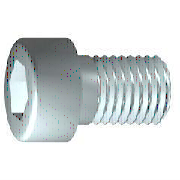
# Autodesk Inventor part: 100021
Saved by Autodesk Inventor 2020.1 (Build 241239000, 239)
## iProperties
Created: 2006-01-26
Part Number: 100021
Material: Steel, Mild
Description: Hexagon Socket Head Cap Screw
Vendor: Autodesk Inc.
Document SubType Name: Modeling
Standard: ISO 4762
Designer: Kevin
Standard Revision: Fourth edition 2004-03-01
Standards Organization: ISO
Language: en-US
Size Designation: M8 x 65
Categories: <MemberInstance><Categories><Category DisplayName="Fasteners" InternalName="e4da775c-781d-43d5-af7c-5136215cf5a6" Mnemonic="FSTN"><Category DisplayName="Bolts" InternalName="536e6df0-f778-49ac-b2f2-25c71d2aa0b2" Mnemonic="SCRW"><CategoryParameter DisplayName="Nominal Diameter" InternalName="8bbe3f8e-44cf-40a9-a251-3a6edc8168d6" Mnemonic="nomdia"/><CategoryParameter DisplayName="Nominal Length" InternalName="238ecbaf-3e6c-45dd-aa95-4068c8e0fd02" Mnemonic="nomlen"/><CategoryParameter DisplayName="Thread Series Designation" InternalName="87c5849c-b3a5-4c3e-9c9b-2feecef9be86" Mnemonic="thrserdsgn"/><CategoryParameter DisplayName="Thread Class" InternalName="ebc0d23b-2cc6-4d2a-b376-d52aae53bab6" Mnemonic="thrclss"/><CategoryParameter DisplayName="Thread Designation" InternalName="586d5e89-370a-4089-914f-0110033585c7" Mnemonic="thrdesign"/><CategoryParameter DisplayName="Thread Type" InternalName="b4bbb7bc-d6aa-4c9f-a9a9-4152b9f6fe49" Mnemonic="thrtype"/><CategoryParameter DisplayName="Threads per Unit" InternalName="bdc6e7d2-ffd0-4d9c-a173-16b95ebb912d" Mnemonic="thrperunit1"/><CategoryParameter DisplayName="Thread Pitch" InternalName="bb82302e-82d8-4176-8fc1-c5d7bb17d5ad" Mnemonic="pitch1"/><CategoryParameter DisplayName="Nominal Diameter Designation" InternalName="03caf894-eafd-4c09-a035-916ac084b87b" Mnemonic="nomdiadesig"/><Category DisplayName="Socket Head" InternalName="55e06bf3-7e58-486c-bbdc-745fcc60664d" Mnemonic="CLSCRW"><CategoryParameter DisplayName="Shank Diameter" InternalName="179dbae3-102f-48bb-85fe-1e3ecd34f7cc" Mnemonic="grpdia"/><CategoryParameter DisplayName="Grip Length" InternalName="52eab69f-422f-4795-9995-175a1b827e67" Mnemonic="grplen"/><CategoryParameter DisplayName="Thread Length" InternalName="3268731d-5f9a-4750-8b01-4a959c46fbf2" Mnemonic="thrlen"/><CategoryParameter DisplayName="Head Diameter" InternalName="46177176-dbdd-4a1b-aefd-4c60c45016af" Mnemonic="headdia"/><CategoryParameter DisplayName="Head Height" InternalName="99c92c4c-4a02-4ebe-9e64-948fb169e19e" Mnemonic="headh"/><CategoryParameter DisplayName="Type" InternalName="59a7e495-7a0c-4a5c-bdfd-c090c5f6e2db" Mnemonic="type"/></Category></Category></Category></Categories><FamilyTemplate Id="si0145"><FamilyTemplateParameters><FamilyTemplateParameter ObjectType="kUserParameterObject" ValueType="xs:double" Id="1" ObjectReferenceKey="GUL"/><FamilyTemplateParameter ObjectType="kUserParameterObject" ValueType="xs:double" Id="2" ObjectReferenceKey="SPD"/><FamilyTemplateParameter ObjectType="kUserParameterObject" ValueType="xs:double" Id="3" ObjectReferenceKey="NLG"/><FamilyTemplateParameter ObjectType="kUserParameterObject" ValueType="xs:double" Id="4" ObjectReferenceKey="KOD"/><FamilyTemplateParameter ObjectType="kUserParameterObject" ValueType="xs:double" Id="5" ObjectReferenceKey="TOA"/><FamilyTemplateParameter ObjectType="kUserParameterObject" ValueType="xs:double" Id="6" ObjectReferenceKey="GD1"/><FamilyTemplateParameter ObjectType="kUserParameterObject" ValueType="xs:double" Id="7" ObjectReferenceKey="GEL"/><FamilyTemplateParameter ObjectType="kUserParameterObject" ValueType="xs:double" Id="8" ObjectReferenceKey="SW"/><FamilyTemplateParameter ObjectType="kUserParameterObject" ValueType="xs:double" Id="9" ObjectReferenceKey="THREADDIA"/><FamilyTemplateParameter ObjectType="kUserParameterObject" ValueType="xs:double" Id="10" ObjectReferenceKey="INTI"/><FamilyTemplateParameter ObjectType="kUserParameterObject" ValueType="xs:double" Id="11" ObjectReferenceKey="BDM"/><FamilyTemplateParameter ObjectType="kUserParameterObject" ValueType="xs:double" Id="12" ObjectReferenceKey="FAWI"/><FamilyTemplateParameter ObjectType="kUserParameterObject" ValueType="xs:double" Id="13" ObjectReferenceKey="RR"/><FamilyTemplateParameter ObjectType="kUserParameterObject" ValueType="xs:double" Id="14" ObjectReferenceKey="KOH"/><FamilyTemplateParameter ObjectType="kUserParameterObject" ValueType="xs:double" Id="15" ObjectReferenceKey="TPU"/><FamilyTemplateParameter ObjectType="kUserParameterObject" ValueType="xs:double" Id="16" ObjectReferenceKey="PTC"/><FamilyTemplateParameter ObjectType="kUserParameterObject" ValueType="xs:double" Id="17" ObjectReferenceKey="NND"/><FamilyTemplateParameter ObjectType="kUserParameterObject" ValueType="xs:double" Id="18" ObjectReferenceKey="GD"/><FamilyTemplateParameter ObjectType="kUserParameterObject" ValueType="xs:double" Id="19" ObjectReferenceKey="GAL"/><FamilyTemplateParameter ObjectType="kUserParameterObject" ValueType="xs:double" Id="20" ObjectReferenceKey="E0"/><FamilyTemplateParameter ObjectType="kPropertyObject" ValueType="xs:string" Id="100" ObjectReferenceKey="{32853F0F-3444-11D1-9E93-0060B03C1CA6}" SubObjectId="52"/><FamilyTemplateParameter ObjectType="kPropertyObject" ValueType="xs:string" Id="101" ObjectReferenceKey="{32853F0F-3444-11D1-9E93-0060B03C1CA6}" SubObjectId="49"/><FamilyTemplateParameter ObjectType="kPropertyObject" ValueType="xs:string" Id="102" ObjectReferenceKey="{32853F0F-3444-11D1-9E93-0060B03C1CA6}" SubObjectId="37"/><FamilyTemplateParameter ObjectType="kPropertyObject" ValueType="xs:string" Id="103" ObjectReferenceKey="{32853F0F-3444-11D1-9E93-0060B03C1CA6}" SubObjectId="47"/><FamilyTemplateParameter ObjectType="kPropertyObject" ValueType="xs:string" Id="104" ObjectReferenceKey="{32853F0F-3444-11D1-9E93-0060B03C1CA6}" SubObjectId="48"/><FamilyTemplateParameter ObjectType="kPropertyObject" ValueType="xs:string" Id="105" ObjectReferenceKey="{32853F0F-3444-11D1-9E93-0060B03C1CA6}" SubObjectId="5"/><FamilyTemplateParameter ObjectType="kPropertyObject" ValueType="xs:string" Id="106" ObjectReferenceKey="{32853F0F-3444-11D1-9E93-0060B03C1CA6}" SubObjectId="29"/><FamilyTemplateParameter ObjectType="kPropertyObject" ValueType="xs:string" Id="107" ObjectReferenceKey="{32853F0F-3444-11D1-9E93-0060B03C1CA6}" SubObjectId="20"/><FamilyTemplateParameter ObjectType="kPropertyObject" ValueType="xs:string" Id="108" ObjectReferenceKey="{B9600981-DEE8-4547-8D7C-E525B3A1727A}" SubObjectId="17"/><FamilyTemplateParameter ObjectType="kPropertyObject" ValueType="xs:string" Id="109" ObjectReferenceKey="{B9600981-DEE8-4547-8D7C-E525B3A1727A}" SubObjectId="19"/><FamilyTemplateParameter ObjectType="kPropertyObject" ValueType="xs:string" Id="110" ObjectReferenceKey="{B9600981-DEE8-4547-8D7C-E525B3A1727A}" SubObjectId="21"/><FamilyTemplateParameter ObjectType="kPropertyObject" ValueType="xs:string" Id="111" ObjectReferenceKey="{B9600981-DEE8-4547-8D7C-E525B3A1727A}" SubObjectId="9"/><FamilyTemplateParameter ObjectType="kPartDocumentObject" ValueType="xs:string" Id="112" ObjectReferenceKey="" SubObjectId="DisplayName"/><FamilyTemplateParameter ObjectType="kThreadFeatureObject" ValueType="xs:structure" Id="300" ObjectReferenceKey="1002000010000000a2070000000000008000000000000000" SubObjectId="ThreadInfo"><FamilyTemplateParameter ValueType="xs:string" Id="301" SubObjectId="ThreadDesignation"/><FamilyTemplateParameter ValueType="xs:string" Id="302" SubObjectId="ThreadType"/><FamilyTemplateParameter ValueType="xs:string" Id="303" SubObjectId="ThreadClass"/></FamilyTemplateParameter><FamilyTemplateParameter ObjectType="kPartFeatureObject" ValueType="xs:string" Id="400" ObjectReferenceKey="1002000010000000e6050000000000008000000000000000" SubObjectId="Name"/><FamilyTemplateParameter ObjectType="kPartFeatureObject" ValueType="xs:string" Id="401" ObjectReferenceKey="100200001000000095060000000000008000000000000000" SubObjectId="Name"/><FamilyTemplateParameter ObjectType="kPartFeatureObject" ValueType="xs:string" Id="402" ObjectReferenceKey="10020000100000003f0a0000000000008000000000000000" SubObjectId="Name"/><FamilyTemplateParameter ObjectType="kPartFeatureObject" ValueType="xs:string" Id="403" ObjectReferenceKey="1002000010000000a2070000000000008000000000000000" SubObjectId="Name"/><FamilyTemplateParameter ObjectType="kPartFeatureObject" ValueType="xs:string" Id="404" ObjectReferenceKey="10020000100000004b080000000000008000000000000000" SubObjectId="Name"/><FamilyTemplateParameter ObjectType="kPartFeatureObject" ValueType="xs:string" Id="405" ObjectReferenceKey="10020000100000001b000000000000008000000000000000" SubObjectId="Name"/><FamilyTemplateParameter ObjectType="kPartFeatureObject" ValueType="xs:string" Id="406" ObjectReferenceKey="100200001000000008060000000000008000000000000000" SubObjectId="Name"/><FamilyTemplateParameter ObjectType="kiMateDefinitionObject" ValueType="xs:string" Id="500" ObjectReferenceKey="040101001000000056c3c3acc3436235c70bd6913be2b3c4" SubObjectId="Name"/><FamilyTemplateParameter ObjectType="kiMateDefinitionObject" ValueType="xs:string" Id="501" ObjectReferenceKey="0401010010000000e313b551ae4b9e8382ff6e817fb601cd" SubObjectId="Name"/><FamilyTemplateParameter ObjectType="kiMateDefinitionObject" ValueType="xs:string" Id="502" ObjectReferenceKey="040101001000000034281a2f2942eb86b29cb3a32be18ec1" SubObjectId="Name"/><FamilyTemplateParameter ObjectType="kiPartTableColumnObject" ValueType="xs:string" Id="503" ObjectReferenceKey="RID"/><FamilyTemplateParameter ObjectType="kiPartTableColumnObject" ValueType="xs:string" Id="504" ObjectReferenceKey="DACOOKIE"/><FamilyTemplateParameter ObjectType="kiPartTableColumnObject" ValueType="xs:string" Id="505" ObjectReferenceKey="KLG"/><FamilyTemplateParameter ObjectType="kiPartTableColumnObject" ValueType="xs:string" Id="506" ObjectReferenceKey="THREADCLASSEXT"/><FamilyTemplateParameter ObjectType="kiPartTableColumnObject" ValueType="xs:string" Id="507" ObjectReferenceKey="SIZE_SEL"/><FamilyTemplateParameter ObjectType="kiPartTableColumnObject" ValueType="xs:string" Id="508" ObjectReferenceKey="THREADTYPE"/></FamilyTemplateParameters></FamilyTemplate><CategoryParameterMap><ParamToTemplateMap><ParamToTemplate CategoryParameter="//CategoryParameter[@InternalName='179dbae3-102f-48bb-85fe-1e3ecd34f7cc']" TemplateParameter="11"/><ParamToTemplate CategoryParameter="//CategoryParameter[@InternalName='316934ee-8fe1-4c7a-9c36-f2d79e1add1a']" TemplateParameter="504"/><ParamToTemplate CategoryParameter="//CategoryParameter[@InternalName='2675968c-4ce5-49e0-a4f5-552d29089031']" TemplateParameter="100"/><ParamToTemplate CategoryParameter="//CategoryParameter[@InternalName='8b46a4cc-9585-4fed-90c3-899f57e09a73']" TemplateParameter="110"/><ParamToTemplate CategoryParameter="//CategoryParameter[@InternalName='3268731d-5f9a-4750-8b01-4a959c46fbf2']" TemplateParameter="7"/><ParamToTemplate CategoryParameter="//CategoryParameter[@InternalName='52eab69f-422f-4795-9995-175a1b827e67']" TemplateParameter="505"/><ParamToTemplate CategoryParameter="//CategoryParameter[@InternalName='46177176-dbdd-4a1b-aefd-4c60c45016af']" TemplateParameter="4"/><ParamToTemplate CategoryParameter="//CategoryParameter[@InternalName='99c92c4c-4a02-4ebe-9e64-948fb169e19e']" TemplateParameter="14"/><ParamToTemplate CategoryParameter="//CategoryParameter[@InternalName='818a152a-d3c3-49ca-80ee-df7d91421b8e']" TemplateParameter="107"/><ParamToTemplate CategoryParameter="//CategoryParameter[@InternalName='238ecbaf-3e6c-45dd-aa95-4068c8e0fd02']" TemplateParameter="3"/><ParamToTemplate CategoryParameter="//CategoryParameter[@InternalName='8bbe3f8e-44cf-40a9-a251-3a6edc8168d6']" TemplateParameter="17"/><ParamToTemplate CategoryParameter="//CategoryParameter[@InternalName='016b6077-bfbe-49bd-92c9-d8d59c39c941']" TemplateParameter="105"/><ParamToTemplate CategoryParameter="//CategoryParameter[@InternalName='bb82302e-82d8-4176-8fc1-c5d7bb17d5ad']" TemplateParameter="16"/><ParamToTemplate CategoryParameter="//CategoryParameter[@InternalName='8e5e0294-fc51-4c8f-b3d7-003dc5ed94f6']" TemplateParameter="503"/><ParamToTemplate CategoryParameter="//CategoryParameter[@InternalName='03caf894-eafd-4c09-a035-916ac084b87b']" TemplateParameter="507"/><ParamToTemplate CategoryParameter="//CategoryParameter[@InternalName='ebc0d23b-2cc6-4d2a-b376-d52aae53bab6']" TemplateParameter="506"/><ParamToTemplate CategoryParameter="//CategoryParameter[@InternalName='586d5e89-370a-4089-914f-0110033585c7']" TemplateParameter="301"/><ParamToTemplate CategoryParameter="//CategoryParameter[@InternalName='b4bbb7bc-d6aa-4c9f-a9a9-4152b9f6fe49']" TemplateParameter="508"/><ParamToTemplate CategoryParameter="//CategoryParameter[@InternalName='bdc6e7d2-ffd0-4d9c-a173-16b95ebb912d']" TemplateParameter="15"/></ParamToTemplateMap></CategoryParameterMap></MemberInstance>
Density: 1 g/cm^3
Appearance: Steel
Author: Kevin
Autodesk Inventor part; units mm, degrees
ref_plane "YZ Plane" through (0, 0, 0) normal (1, 0, 0) x (0, 1, 0)
ref_plane "XZ Plane" through (0, 0, 0) normal (0, 1, 0) x (-1, 0, 0)
sketch "Sketch1" plane through (0, 0, 0) normal (0, 0, 1) x (1, 0, 0)
  line L0 (-2, 0) -> (65, 0)
  line L1 (65, 0) -> (65, 4)
  line L2 (65, 4) -> (37, 4)
  line L3 (37, 4) -> (36.2331, 4)
  line L4 (36.2331, 4) -> (0, 4)
  line L5 (0, 4) -> (0, 6.5)
  line L6 (0, 6.5) -> (-8, 6.5)
  line L7 (-8, 6.5) -> (-8, 3.4641)
  line L8 (-8, 3.4641) -> (-4, 3.4641)
  line L9 (-4, 3.4641) -> (-2, 0)
  line L10 (-15.3, 0) -> (86.9, 0) projected
  line L11 (0, -0.65) -> (0, 8.45) projected
  line L12 (37, 4) -> (0, 4) construction
  dimension "d1" = 28
  dimension "d2" = 0.7669
  dimension "d3" = 8
  dimension "d4" = 4
  dimension "d5" = 60
  dimension "d6" = 8
  dimension "d7" = 8
  dimension "d8" = 6.9282
  dimension "d9" = 13
  dimension "d26" = 65
  constraints: 22 end point, 6 parallel, 2 collinear, 2 perpendicular, 1 horizontal, 1 point on line
  measures "d1" distance from line of L2.end L1
  measures "d2" distance of L3.end L2.end
  measures "d3" distance between parallel lines of L7 L5
  measures "d4" distance of L7.end L8.end
  measures "d5" angle of L9 L0
  measures "d6" diameter of L2 L0
  measures "d7" diameter of L4 L0
  measures "d8" diameter of L8 L0
  measures "d9" diameter of L6 L0
  measures "d26" distance between parallel lines of L11 L1
revolve "Body" add sketch "Sketch1" angle 360 about axis through (-2, 0, 0) along (1, 0, 0)
sketch "Sketch2" plane through (-8, 0, 0) normal (-1, 0, 0) x (0, 0, 1)
  circle A0 centre (0, 0) radius 3.4641 projected
  line L0 (0, -7.8) -> (0, 10.4) projected
  line L1 (-7.8, 0) -> (10.4, 0) projected
  line L2 (3.4641, 0) -> (1.7321, -3)
  line L3 (1.7321, -3) -> (-1.7321, -3)
  line L4 (-1.7321, -3) -> (-3.4641, 0)
  line L5 (-3.4641, 0) -> (-1.7321, 3)
  line L6 (-1.7321, 3) -> (1.7321, 3)
  line L7 (1.7321, 3) -> (3.4641, 0)
  constraints: 12 end point, 1 coincident, 1 horizontal alignment, 1 point on line, 12 other
extrude "Slot" add sketch "Sketch2" against normal up to next contours L7 A0 | A0 L2 | L6 L0 A0 | A0 L0 L3 | L0 L6 A0 | A0 L3 L0 | L4 A0 | A0 L5
fillet "Fillet1" radius 0.8 1 edges at (-8, -6.5, 0)
thread "Thread" size "M8x1.25" class "6g" standard "ISO Metric profile" length 28
chamfer "Chamfer1" distance 0.7668 distance2 0.7668 1 edges at (65, -4, 0) measured on face at (65, -1.1806, -1.575)
ref_plane "Work Plane1" through (29, 0, 0) normal (0, -1, 0) x (1, 0, 0)
equation "\"d1\" = GEL"
equation "\"d3\" = KOH"
equation "\"d4\" = INTI"
equation "\"d6\" = GD"
equation "\"d7\" = BDM"
equation "\"d8\" = 1.1547 * SW"
equation "\"d9\" = KOD"
equation "\"d26\" = NLG"
equation "\"d17\" = RR"
equation "\"d13\" = GEL"
equation "\"d15\" = -0.5 * SPD + 0.5 * GD"
equation "\"d16\" = GUL"
equation "\"GD\" = 8"
equation "\"NLG\" = 65"
equation "\"GEL\" = 28"
equation "\"KOD\" = 13"
equation "\"KOH\" = 8"
equation "\"INTI\" = 4"
equation "\"GAL\" = 0.61345 * PTC"
equation "\"GUL\" = 0.61345 * PTC"
equation "\"BDM\" = NND"
equation "\"SW\" = 6"
equation "\"RR\" = 0.8"
equation "\"SPD\" = NND - 1.2269 * PTC"
equation "\"TOA\" = 30deg"
equation "\"GD1\" = THREADDIA - 1.2269 * PTC"
equation "\"THREADDIA\" = 8"
equation "\"FAWI\" = 45deg"
equation "\"PTC\" = 1.25"
equation "\"NND\" = 8"
equation "\"E0\" = 1.155 * SW"
body "Solid1"
